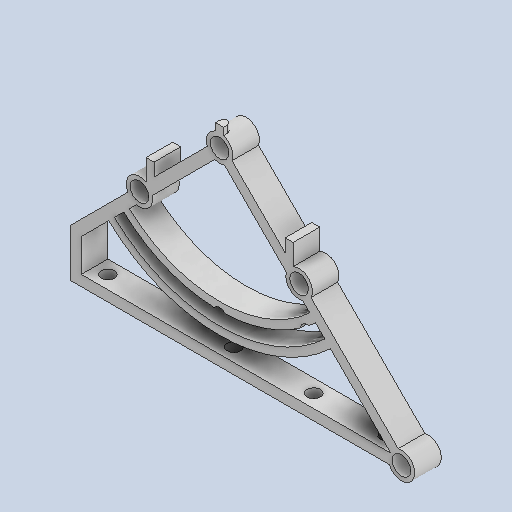
# Autodesk Inventor part: BigCage2
Saved by Autodesk Inventor 2025 (Build 290162000, 162)
## iProperties
Created: 2025-08-07
Part Number: BigCage2
Material: Generic
Document SubType Name: Modeling
Designer: Pravoslav
Density: 1 g/cm^3
Appearance: Default
Author: Pravoslav
Autodesk Inventor part; units mm, degrees
ref_plane "YZ Plane" through (0, 0, 0) normal (1, 0, 0) x (0, 1, 0)
ref_plane "XZ Plane" through (0, 0, 0) normal (0, 1, 0) x (-1, 0, 0)
ref_plane "XY Plane" through (0, 0, 0) normal (0, 0, 1) x (1, 0, 0)
sketch "Sketch1" plane through (0, 0, 0) normal (0, 0, 1) x (1, 0, 0)
  line L0 (-70, 2) -> (70, 2)
  line L1 (70, 2) -> (70, -2)
  line L2 (70, -2) -> (-70, -2)
  line L3 (-70, -2) -> (-70, 2)
  line L4 (-70, 2) -> (70, -2) construction
  line L5 (70, 2) -> (-70, -2) construction
  line L6 (-70, 2) -> (44.4369, 116.4369)
  line L7 (-70, 2) -> (91.8383, 2) construction
  line L8 (70, 2) -> (-21.2026, 93.2026)
  line L9 (-64.3431, 2) -> (2.8284, 69.1716)
  line L10 (-2.8284, 69.1716) -> (64.3431, 2)
  circle A0 centre (0, 69.1716) radius 3.5
  circle A1 centre (0, 69.1716) radius 5
  circle A2 centre (-67.6199, 0) radius 3.5
  circle A3 centre (-67.6199, 0) radius 5
  circle A4 centre (68.3761, 0) radius 3.5
  circle A5 centre (68.3761, 0) radius 5
  circle A6 centre (29.8984, 39.897) radius 3.5
  circle A7 centre (29.8984, 39.897) radius 5
  line L11 (27.6414, 44.3586) -> (-27.6414, 44.3586)
  line L12 (-27.6414, 44.3586) -> (-27.6414, 52.2202)
  line L13 (-27.6414, 52.2202) -> (-24.6414, 52.2202)
  line L14 (-24.6414, 52.2202) -> (-24.6414, 47.3586)
  line L15 (27.6414, 44.3586) -> (27.6414, 52.2202)
  line L16 (27.6414, 52.2202) -> (24.6414, 52.2202)
  line L17 (24.6414, 52.2202) -> (24.6414, 47.3586)
  circle A8 centre (0, 69.1716) radius 50
  circle A9 centre (0, 69.1716) radius 53
  circle A10 centre (0, 69.1716) radius 58
  circle A11 centre (0, 69.1716) radius 61
  arc A12 (2.1548, 16.1686) -> (-2.1058, 16.2485) centre (-0.005, 14.6373) ccw
  arc A13 (33.4747, 28.0809) -> (30.3172, 25.699) centre (32.9561, 25.4847) ccw
  line L18 (-2.1058, 16.2485) -> (-2.1315, 16.2145)
  line L19 (-0.1162, 2) -> (-0.1162, -3.5)
  circle A14 centre (-30.1308, 39.897) radius 3.5
  circle A15 centre (-30.1308, 39.897) radius 5
  line L20 (-70.2324, 2) -> (69.7676, -2) construction
  circle A16 centre (-30.1308, 39.897) radius 3.5
  circle A17 centre (-30.1308, 39.897) radius 5
  line L21 (-56, -2) -> (-56, 16)
  line L22 (-52, 20) -> (-52, -2)
  point P0 (0, 0)
  point P1 (1.8262, 64.517)
  point P2 (25.0868, 41.2564)
  point P3 (31.2578, 35.0853)
  point P4 (64.3431, 2)
  point P5 (-1.8262, 64.517)
  point P6 (-4.6546, 67.3454)
  point P7 (-67.0344, 4.9656)
  point P8 (-63.0374, -2)
  point P9 (63.7935, -2)
  point P10 (67.1521, 4.8479)
  point P11 (34.36, 37.64)
  point P12 (4.6546, 67.3454)
  point P13 (-41.6961, 24.647)
  point P14 (41.6961, 24.647)
  point P15 (39.5736, 26.7696)
  point P16 (-39.5736, 26.7696)
  point P17 (-36.0358, 30.3074)
  point P18 (36.0358, 30.3074)
  point P19 (33.9128, 32.4303)
  point P20 (-33.9128, 32.4303)
  point P21 (2.1218, 16.2141)
  point P22 (-31.3061, 35.0371)
  point P23 (-25.2709, 41.0722)
  point P24 (-27.7217, 44.2783)
  point P25 (-34.5122, 37.4878)
  point P26 (-56, 7)
  point P27 (-52, 2)
  point P28 (-52, 14.3431)
  point P29 (-56, 10.3431)
  point P30 (-56, 2)
  dimension "d16" = 10
  dimension "d0" = 140
  dimension "d1" = 4
  dimension "d2" = 45
  dimension "d3" = 4
  dimension "d6" = 4
  dimension "d7" = 4
  dimension "d8" = 4
  dimension "d9" = 7
  dimension "d10" = 10
  dimension "d11" = 7
  dimension "d12" = 10
  dimension "d13" = 7
  dimension "d14" = 10
  dimension "d15" = 7
  dimension "d17" = 3
  dimension "d18" = 3
  dimension "d21" = 3
  dimension "d22" = 3
  dimension "d23" = 5
  dimension "d24" = 100
  dimension "d42" = 4
  dimension "d43" = 14
  constraints: 46 end point, 17 centre point, 15 point on line, 10 coincident, 7 perpendicular, 7 point on circle, 6 symmetric about line, 3 horizontal, 3 midpoint, 3 parallel, 2 vertical, 1 equal length, 7 other
  measures "d0" distance of L1.end L2.end
  measures "d1" distance between parallel lines of L0 L2
  measures "d2" angle of L7 L6
  measures "d3" distance from line of L9.end L6
  measures "d6" distance from line of L6 L9.start
  measures "d7" distance from line of L10.start L8
  measures "d8" distance from line of L10 L0.end
  measures "d9" diameter of A0
  measures "d10" diameter of A1
  measures "d11" diameter of A2
  measures "d12" diameter of A3
  measures "d13" diameter of A4
  measures "d14" diameter of A5
  measures "d15" diameter of A6
  measures "d17" distance of L12.end L13.end
  measures "d18" distance of L15.end L16.end
  measures "d21" radial gap between concentric circles of A9 A8
  measures "d22" radial gap between concentric circles of A11 A10
  measures "d23" radial gap between concentric circles of A9 A10
  measures "d24" diameter of A8
  measures "d42" distance from line of point (-56, 7) L22
  measures "d43" distance between parallel lines of L3 L21
extrude "Extrusion1" add sketch "Sketch1" along normal blind 10 contours L6 L22 L9 L21 | L21 L9 L22 L0 | L0 L22 L2 L21 | L6 A11 L9 L22 | L0 L19 L2 L22 | L6 A10 L9 A11 | L0 A5 L2 L19 | L9 A10 L10 A11 | L6 A9 L9 A10 | L0 A4 L2 A5 | A11 L8 A5 L10 | L10 A10 L8 A11 | L2 A4 L8 A5 | L6 A8 L9 A9 | L10 A5 L8 A4 L0 | L9 A8 L10 A9 A13 A12 L18 | L10 A9 L8 A10 | L6 A15 L9 A8 | L10 A8 L8 A9 | A15 L6 A14 | L6 A14 L9 A15 | L9 A14 A15 | L10 A7 L8 A8 | A15 L9 A14 L6 | L6 L11 L9 A15 | A1 L8 A0 L6 | L6 A0 L8 A1 | A7 L10 A6 | L10 A6 L8 A7 | L12 L13 L14 L6 | L6 A1 L9 L11 | L8 A0 L6 A1 | A7 L8 A6 L10 | L10 L11 A7 | L8 A6 A7 | A1 L10 A0 L8 | L8 L11 L10 A1 | L6 A0 L9 A1 | L8 L17 L16 L15 | L9 A0 L10 A1
extrude "Extrusion2" cut sketch "Sketch1" along normal blind 10 contours L18 A12 A9 | A9 A13
sketch "Sketch2" plane through (0, 0, 10) normal (0, 0, 1) x (1, 0, 0)
  line L0 (-1.5, 73.6716) -> (-1.5, 76.6716)
  line L1 (-1.5, 76.6716) -> (1.5, 76.6716)
  line L2 (1.5, 76.6716) -> (1.5, 73.6716)
  arc A0 (4.6546, 67.3454) -> (-4.6546, 67.3454) centre (0, 69.1716) ccw projected
  line L3 (-1.5, 73.6716) -> (1.5, 73.6716)
  circle A1 centre (0, 69.1716) radius 3.5 projected
  point P0 (0, 0)
  point P1 (0, 74.1716)
  point P2 (-1.5, 73.9413)
  point P3 (1.5, 73.9413)
  dimension "d27" = 3
  dimension "d28" = 1.5
  dimension "d31" = 3
  dimension "d32" = 1
  constraints: 8 end point, 2 perpendicular, 1 horizontal, 1 point on circle, 1 vertical
  measures "d27" distance of L0.end L1.end
  measures "d28" distance from line of point (0, 74.172) L0
  measures "d31" distance between parallel lines of L3 L1
  measures "d32" distance edge to line of A1 L3
extrude "Extrusion3" add sketch "Sketch2" against normal blind 3 contours L0 L1 L2 A0
fillet "Fillet1" radius 1.5 2 edges at (1.5, 75.3064, 7) (-1.5, 75.3064, 7)
sketch "Sketch3" plane through (-70, -2, 0) normal (0, -1, 0) x (1, 0, 0)
  line L0 (134.3431, 0) -> (134.3431, 10) projected
  line L1 (5.6569, 0) -> (5.6569, 10) projected
  circle A0 centre (23, 5) radius 2.5
  circle A1 centre (128, 5) radius 2.5
  line L2 (140, 0) -> (140, 10) projected
  line L3 (14, 10) -> (133.7935, 10) projected
  point P0 (70, 0)
  point P1 (0, 10)
  dimension "d34" = 5
  dimension "d35" = 5
  dimension "d36" = 105
  dimension "d37" = 12
  dimension "d38" = 5
  dimension "d39" = 5
  constraints: 2 centre point
  measures "d34" diameter of A0
  measures "d35" diameter of A1
  measures "d36" distance of A1.centre A0.centre
  measures "d37" distance from line of L2 A1.centre
  measures "d38" distance from line of L3 A1.centre
  measures "d39" distance from line of L3 A0.centre
extrude "Extrusion4" cut sketch "Sketch3" against normal up to surface (4 mm away)
sketch "Sketch4" plane through (-56, -2, 0) normal (0, -1, 0) x (1, 0, 0)
  circle A0 centre (86.3685, 5) radius 2.5
  circle A1 centre (56.3685, 5) radius 2.5
  line L0 (0, 0) -> (119.7935, 0) projected
  line L1 (53.8942, 0) -> (58.1218, 0) projected
  line L2 (53.8942, 10) -> (58.1218, 10) projected
  line L3 (53.8685, 0) -> (53.8685, 10) projected
  point P0 (56, 0)
  dimension "d44" = 5
  dimension "d45" = 5
  dimension "d46" = 5
  dimension "d47" = 5
  dimension "d48" = 30
  dimension "d49" = 2.5
  constraints: 2 centre point
  measures "d44" diameter of A0
  measures "d45" diameter of A1
  measures "d46" distance from line of L0 A0.centre
  measures "d47" distance from line of L0 A1.centre
  measures "d48" distance of A1.centre A0.centre
  measures "d49" distance from line of L3 A1.centre
extrude "Extrusion5" cut sketch "Sketch4" against normal up to surface (4 mm away)
body "Solid1"
